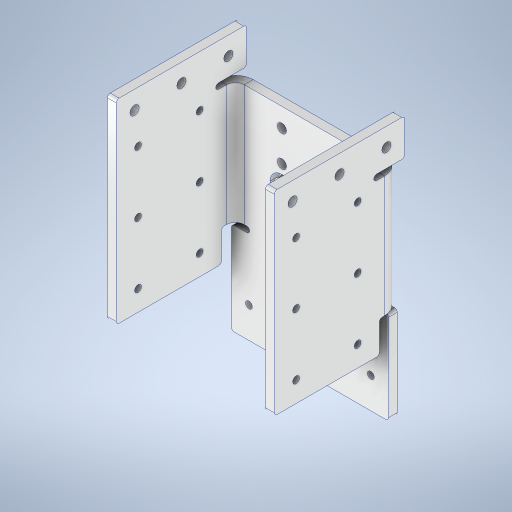
# Autodesk Inventor part: Printhead Baseplate
Saved by Autodesk Inventor 2024 (Build 280153000, 153)
## iProperties
Created: 2025-01-03
Part Number: Printhead Baseplate
Material: Aluminum 6061
Document SubType Name: Sheet Metal
Designer: Ishaan
Density: 2.7 g/cm^3
Sheet Metal Rule: SendCutSend_1-8_Alu
Appearance: Aluminum - Flat
Flat Pattern Width: 13.9913 cm
Flat Pattern Length: 9.325 cm
Flat Pattern Area: 130.469 cm^2
Sheet Metal Width: 139.913 mm
Sheet Metal Length: 93.250 mm
Sheet Metal Area: 13046.921 mm^2
Author: Ishaan
Autodesk Inventor part; units mm, degrees
ref_plane "YZ Plane" through (0, 0, 0) normal (1, 0, 0) x (0, 1, 0)
ref_plane "XZ Plane" through (0, 0, 0) normal (0, 1, 0) x (-1, 0, 0)
ref_plane "XY Plane" through (0, 0, 0) normal (0, 0, 1) x (1, 0, 0)
sketch "Sketch1" plane through (0, 0, 0) normal (0, 0, 1) x (1, 0, 0)
  line L0 (28, -13.5) -> (-28, -13.5)
  line L1 (-28, -13.5) -> (-28, 13.5)
  line L2 (-28, 13.5) -> (28, 13.5)
  line L3 (28, 13.5) -> (28, -13.5)
  line L4 (28, -13.5) -> (-28, 13.5) construction
  line L5 (-28, -13.5) -> (28, 13.5) construction
  line L6 (-28, -13.5) -> (28, -13.5)
  line L7 (28, -13.5) -> (28, -46.5)
  line L8 (28, -46.5) -> (-28, -46.5)
  line L9 (-28, -46.5) -> (-28, -13.5)
  line L10 (10, -10) -> (-10, -10) construction
  line L11 (-10, -10) -> (-10, 10) construction
  line L12 (-10, 10) -> (10, 10) construction
  line L13 (10, 10) -> (10, -10) construction
  line L14 (10, -10) -> (-10, 10) construction
  line L15 (-10, -10) -> (10, 10) construction
  line L16 (28, -47) -> (-28, -47) construction
  line L17 (-28, -47) -> (-28, -17) construction
  line L18 (-28, -17) -> (28, -17) construction
  line L19 (28, -17) -> (28, -47) construction
  line L20 (28, -47) -> (-28, -17) construction
  line L21 (-28, -47) -> (28, -17) construction
  circle A0 centre (0, -32) radius 11 construction
  circle A1 centre (0, -32) radius 8 construction
  line L22 (5.6569, -37.6569) -> (-5.6569, -37.6569) construction
  line L23 (-5.6569, -37.6569) -> (-5.6569, -26.3431) construction
  line L24 (-5.6569, -26.3431) -> (5.6569, -26.3431) construction
  line L25 (5.6569, -26.3431) -> (5.6569, -37.6569) construction
  line L26 (5.6569, -37.6569) -> (-5.6569, -26.3431) construction
  line L27 (-5.6569, -37.6569) -> (5.6569, -26.3431) construction
  line L28 (-21.75, -32) -> (21.75, -32) construction
  line L29 (16, -16) -> (-16, -16)
  line L30 (-16, -16) -> (-16, 16)
  line L31 (-16, 16) -> (16, 16)
  line L32 (16, 16) -> (16, -16)
  line L33 (16, -16) -> (-16, 16) construction
  line L34 (-16, -16) -> (16, 16) construction
  line L35 (16, -47) -> (-16, -47) construction
  line L36 (-16, -47) -> (-16, -17) construction
  line L37 (-16, -17) -> (16, -17) construction
  line L38 (16, -17) -> (16, -47) construction
  line L39 (16, -47) -> (-16, -17) construction
  line L40 (-16, -47) -> (16, -17) construction
  line L41 (13, -38.5) -> (-13, -38.5) construction
  line L42 (-13, -38.5) -> (-13, -25.5) construction
  line L43 (-13, -25.5) -> (13, -25.5) construction
  line L44 (13, -25.5) -> (13, -38.5) construction
  line L45 (13, -38.5) -> (-13, -25.5) construction
  line L46 (-13, -38.5) -> (13, -25.5) construction
  line L47 (28, -21) -> (-28, -21)
  line L48 (-28, -21) -> (-28, -43)
  line L49 (-28, -43) -> (28, -43)
  line L50 (28, -43) -> (28, -21)
  line L51 (28, -21) -> (-28, -43) construction
  line L52 (-28, -21) -> (28, -43) construction
  line L53 (-28, 13.5) -> (28, 13.5)
  line L54 (28, 13.5) -> (28, 35.25)
  line L55 (28, 35.25) -> (-28, 35.25)
  line L56 (-28, 35.25) -> (-28, 13.5)
  point P0 (0, 0)
  point P1 (-16, 13.5)
  point P2 (16, 13.5)
  point P3 (-28, -43)
  point P4 (28, -43)
  dimension "d8" = 16
  dimension "d0" = 56
  dimension "d1" = 27
  dimension "d2" = 60
  dimension "d3" = 20
  dimension "d4" = 20
  dimension "d5" = 30
  dimension "d6" = 32
  dimension "d7" = 22
  dimension "d9" = 43.5
  dimension "d32" = 32
  dimension "d33" = 32
  dimension "d41" = 32
  dimension "d42" = 26
  dimension "d43" = 13
  dimension "d61" = 22
  dimension "d73" = 35.25
  constraints: 114 end point, 20 parallel, 17 midpoint, 16 coincident, 11 horizontal, 11 perpendicular, 3 collinear, 2 point on line, 1 centre point, 1 vertical alignment, 3 other
  measures "d0" distance of L1.end L2.end
  measures "d1" distance of L0.end L1.end
  measures "d2" distance between parallel lines of L8 L2
  measures "d3" distance of L11.end L12.end
  measures "d4" distance of L10.end L11.end
  measures "d5" distance of L16.end L17.end
  measures "d6" distance of point (0, -32) point (0, 0)
  measures "d7" diameter of A0
  measures "d9" distance of L28.start L28.end
  measures "d32" distance of L30.end L31.end
  measures "d33" distance of L29.end L30.end
  measures "d41" distance of L36.end L37.end
  measures "d42" distance of L42.end L43.end
  measures "d43" distance of L41.end L42.end
  measures "d61" distance between parallel lines of L49 L47
  measures "d73" distance from line of L55 point (0, 0)
sketch "Sketch15" plane through (0, 0, 0) normal (0, 0, -1) x (-1, 0, 0)
  arc A0 (-13, -10) -> (-10, -13) centre (-10, -10) ccw projected
  line L0 (-10, -13) -> (10, -13) projected
  arc A1 (10, -13) -> (13, -10) centre (10, -10) ccw projected
  line L1 (13, -10) -> (13, 10) projected
  arc A2 (13, 10) -> (10, 13) centre (10, 10) ccw projected
  line L2 (10, 13) -> (8.25, 13) projected
  arc A3 (8.25, 14.5) -> (8.25, 13) centre (8.25, 13.75) ccw projected
  line L3 (8.25, 14.5) -> (10, 14.5) projected
  arc A4 (14.5, 10) -> (10, 14.5) centre (10, 10) ccw projected
  line L4 (14.5, 10) -> (14.5, -10) projected
  arc A5 (10, -14.5) -> (14.5, -10) centre (10, -10) ccw projected
  line L5 (10, -14.5) -> (-10, -14.5) projected
  arc A6 (-14.5, -10) -> (-10, -14.5) centre (-10, -10) ccw projected
  line L6 (-14.5, -10) -> (-14.5, 10) projected
  arc A7 (-10, 14.5) -> (-14.5, 10) centre (-10, 10) ccw projected
  line L7 (-10, 14.5) -> (-8.25, 14.5) projected
  arc A8 (-8.25, 13) -> (-8.25, 14.5) centre (-8.25, 13.75) ccw projected
  line L8 (-8.25, 13) -> (-10, 13) projected
  arc A9 (-10, 13) -> (-13, 10) centre (-10, 10) ccw projected
  line L9 (-13, 10) -> (-13, -10) projected
  arc A10 (9.25, 48.736) -> (7.25, 50.736) centre (7.25, 48.736) ccw projected
  line L10 (-7.25, 50.736) -> (7.25, 50.736) projected
  arc A11 (-7.25, 50.736) -> (-9.25, 48.736) centre (-7.25, 48.736) ccw projected
  line L11 (-9.25, 48.736) -> (-9.25, 39.736) projected
  arc A12 (-11.25, 37.736) -> (-9.25, 39.736) centre (-11.25, 39.736) ccw projected
  line L12 (-11.25, 37.736) -> (-23.45, 37.736) projected
  line L13 (-23.45, 37.736) -> (-23.45, -8) projected
  line L14 (-23.45, -8) -> (-22.5, -8) projected
  arc A13 (-22.5, -10) -> (-22.5, -8) centre (-22.5, -9) ccw projected
  line L15 (-22.5, -10) -> (-26, -10) projected
  arc A14 (-26, -10) -> (-28, -12) centre (-26, -12) ccw projected
  line L16 (-28, -41) -> (-28, -12) projected
  arc A15 (-28, -41) -> (-26, -43) centre (-26, -41) ccw projected
  line L17 (26, -43) -> (-26, -43) projected
  arc A16 (26, -43) -> (28, -41) centre (26, -41) ccw projected
  line L18 (28, -12) -> (28, -41) projected
  arc A17 (28, -12) -> (26, -10) centre (26, -12) ccw projected
  line L19 (26, -10) -> (22.5, -10) projected
  arc A18 (22.5, -8) -> (22.5, -10) centre (22.5, -9) ccw projected
  line L20 (22.5, -8) -> (23.45, -8) projected
  line L21 (23.45, -8) -> (23.45, 37.736) projected
  line L22 (23.45, 37.736) -> (11.25, 37.736) projected
  arc A19 (9.25, 39.736) -> (11.25, 37.736) centre (11.25, 39.736) ccw projected
  line L23 (9.25, 39.736) -> (9.25, 48.736) projected
  circle A20 centre (10, 10) radius 1.65 projected
  circle A21 centre (10, -10) radius 1.65 projected
  circle A22 centre (-10, 10) radius 1.65 projected
  circle A23 centre (-10, -10) radius 1.65 projected
  circle A24 centre (5.6569, -26.3431) radius 1.35 projected
  circle A25 centre (-5.6569, -26.3431) radius 1.35 projected
  circle A26 centre (-5.6569, -37.6569) radius 1.35 projected
  circle A27 centre (5.6569, -37.6569) radius 1.35 projected
  circle A28 centre (21.75, -32) radius 1.2295 projected
  circle A29 centre (-21.75, -32) radius 1.2295 projected
  circle A30 centre (0, -32) radius 2.15 projected
  circle A31 centre (10, 28.5) radius 1.65 projected
  circle A32 centre (-10, 28.5) radius 1.65 projected
  circle A33 centre (-10, 17.5) radius 1.65 projected
  circle A34 centre (10, 17.5) radius 1.65 projected
  circle A35 centre (-6, 39.736) radius 1.65 projected
  circle A36 centre (6, 39.736) radius 1.65 projected
  circle A37 centre (6, 47.736) radius 1.65 projected
  circle A38 centre (-6, 47.736) radius 1.65 projected
  circle A39 centre (0, -32) radius 11
  point P0 (0, 0)
  dimension "d145" = 22
  constraints: 1 centre point, 1 coincident
  measures "d145" diameter of A39
extrude "Plate1" add sketch "Sketch1" along normal blind 3.175 contours L7 L47 L9 L0 L30 L29 L32 | L0 L32 L2 L3 | L32 L29 L30 L0 | L0 L30 L2 L32 | L2 L32 L31 L30 L56 L55 L54 | L7 L49 L9 L47 | L0 L1 L2 L30 | L2 L30 L31 L32
hole "Hole1" at (-10, 10, 0) at (-10, -10, 0) at (10, 10, 0) at (10, -10, 0) direction (0, 0, 1) diameter 3.3 end through all
hole "Hole2" at (-5.6569, -26.3431, 0) at (5.6569, -26.3431, 0) at (5.6569, -37.6569, 0) at (-5.6569, -37.6569, 0) direction (0, 0, 1) diameter 2.7 end through all
hole "Hole3" at (-21.75, -32, 0) at (21.75, -32, 0) direction (0, 0, 1) diameter 2.459 end through all thread size "M3x0.5" class "6H" standard "ANSI Metric M Profile"
hole "Hole4" at (0, -32, 0) direction (0, 0, 1) diameter 4.3 end through all
sketch "Sketch2" plane through (0, 0, 3.175) normal (0, 0, 1) x (1, 0, 0)
  line L0 (10, 17.5) -> (-10, 17.5) construction
  line L1 (-10, 17.5) -> (-10, 28.5) construction
  line L2 (-10, 28.5) -> (10, 28.5) construction
  line L3 (10, 28.5) -> (10, 17.5) construction
  line L4 (10, 17.5) -> (-10, 28.5) construction
  line L5 (-10, 17.5) -> (10, 28.5) construction
  point P0 (0, 0)
  point P1 (0, 23)
  dimension "d51" = 20
  dimension "d52" = 11
  dimension "d137" = 23
  constraints: 12 end point, 4 coincident, 2 midpoint, 2 parallel, 1 horizontal, 1 perpendicular, 1 vertical alignment
  measures "d51" distance of L1.end L2.end
  measures "d52" distance of L0.end L1.end
  measures "d137" distance of point (0, 0) point (0, 23)
hole "Hole6" at (-10, 28.5, 3.175) at (10, 28.5, 3.175) at (10, 17.5, 3.175) at (-10, 17.5, 3.175) direction (0, 0, -1) diameter 3.3 end through all
sketch "Sketch8" plane through (0, 0, 3.175) normal (0, 0, 1) x (1, 0, 0)
  circle A0 centre (-10, 17.5) radius 1.65 construction
  circle A1 centre (10, 17.5) radius 1.65 construction
  circle A2 centre (10, 28.5) radius 1.65 construction
  circle A3 centre (-10, 28.5) radius 1.65 construction
  circle A4 centre (0, -32) radius 2.15 construction
  circle A5 centre (21.75, -32) radius 1.2295 construction
  circle A6 centre (-21.75, -32) radius 1.2295 construction
  circle A7 centre (-5.6569, -37.6569) radius 1.35 construction
  circle A8 centre (5.6569, -37.6569) radius 1.35 construction
  circle A9 centre (5.6569, -26.3431) radius 1.35 construction
  circle A10 centre (-5.6569, -26.3431) radius 1.35 construction
  circle A11 centre (10, -10) radius 1.65 construction
  circle A12 centre (10, 10) radius 1.65 construction
  circle A13 centre (-10, -10) radius 1.65 construction
  circle A14 centre (-10, 10) radius 1.65 construction
  line L0 (-28, -43) -> (-28, 35.25) projected
  line L1 (28, -43) -> (-28, -43) projected
  line L2 (28, 35.25) -> (28, -43) projected
  line L3 (-28, 35.25) -> (28, 35.25) projected
  line L4 (-28, -9) -> (-22.5, -9) construction
  line L5 (-28, -10) -> (-22.5, -10)
  line L6 (-22.5, -8) -> (-28, -8)
  arc A15 (-28, -8) -> (-28, -10) centre (-28, -9) ccw
  arc A16 (-22.5, -10) -> (-22.5, -8) centre (-22.5, -9) ccw
  line L7 (28, -9) -> (22.5, -9) construction
  line L8 (28, -8) -> (22.5, -8)
  line L9 (22.5, -10) -> (28, -10)
  arc A17 (28, -10) -> (28, -8) centre (28, -9) ccw
  arc A18 (22.5, -8) -> (22.5, -10) centre (22.5, -9) ccw
  line L10 (-22.5, -9) -> (22.5, -9) construction
  line L11 (-26.625, -8) -> (26.625, -8)
  line L12 (26.625, -8) -> (26.625, 35.25)
  line L13 (26.625, 35.25) -> (-26.625, 35.25)
  line L14 (-26.625, 35.25) -> (-26.625, -8)
  line L15 (-26.625, -8) -> (-29.8, -8) construction
  line L16 (-29.8, -8) -> (-29.8, 35.25) construction
  line L17 (-29.8, 35.25) -> (-26.625, 35.25) construction
  line L18 (-26.625, 35.25) -> (-26.625, -8) construction
  line L19 (26.625, -8) -> (29.8, -8) construction
  line L20 (29.8, -8) -> (29.8, 35.25) construction
  line L21 (29.8, 35.25) -> (26.625, 35.25) construction
  line L22 (26.625, 35.25) -> (26.625, -8) construction
  point P0 (0, 0)
  point P1 (-25.25, -9)
  point P2 (25.25, -9)
  point P3 (0, 35.25)
  point P4 (28, -10)
  point P5 (28, -10)
  point P6 (28, -8)
  point P7 (-28, -8)
  point P8 (-28, -10)
  dimension "d104" = 2
  dimension "d105" = 23
  dimension "d106" = 45
  dimension "d107" = 53.25
  dimension "d108" = 3.175
  constraints: 42 end point, 8 parallel, 8 point on circle, 8 tangent, 6 point on line, 5 perpendicular, 4 centre point, 3 collinear, 3 horizontal, 3 midpoint, 1 equal radius, 1 vertical alignment
  measures "d104" diameter of A16
  measures "d105" distance from line of L4 A4.centre
  measures "d106" distance of L4.end L7.end
  measures "d107" distance between parallel lines of L12 L14
  measures "d108" distance of L16.end L17.end
extrude "Extrusion2" cut sketch "Sketch8" against normal up to surface (3.175 mm away) contours L0 L6 A16 L5 | L0 L3 L14 L6 | L9 A18 L8 L2 | L8 L12 L3 L2
sketch "Sketch9" plane through (-26.625, -8, 3.175) normal (-1, 0, 0) x (0, -1, 0)
  line L0 (-43.25, 0) -> (0, 0)
  line L1 (0, 0) -> (0, 5)
  line L2 (0, 5) -> (-43.25, 5)
  line L3 (-43.25, 5) -> (-43.25, 0)
  constraints: 6 end point, 1 horizontal, 1 perpendicular, 1 vertical
edge flange "Flange3" height 5 angle 90 thickness 3.175 bend radius 3.175 thickness toward (-1, 0, 0) relief straight relief width 2 relief depth 1.5875 corner gap 3.175 corner form 0 edges at (-26.625, 13.625, 3.175) (26.625, 13.625, 3.175) wall of the first edge with corners at (-26.625, 35.25, 3.175) (-26.625, -8, 3.175) (-26.625, -8, 8.175) (-26.625, 35.25, 8.175)
bend "Bend3"
corner "Corner3"
fillet "Fillet2" radius 1 4 edges at (28, -10, 1.5875) (28, -43, 1.5875) (-28, -10, 1.5875) (-28, -43, 1.5875)
sketch "Sketch13" plane through (0, 0, 3.175) normal (0, 0, 1) x (1, 0, 0)
  circle A0 centre (-10, 10) radius 1.65 projected
  circle A1 centre (10, 10) radius 1.65 projected
  circle A2 centre (10, -10) radius 1.65 projected
  circle A3 centre (-10, -10) radius 1.65 projected
  circle A4 centre (-10, 10) radius 3 construction
  circle A5 centre (-10, -10) radius 3 construction
  circle A6 centre (10, -10) radius 3 construction
  circle A7 centre (10, 10) radius 3 construction
  line L0 (10, -13) -> (-10, -13)
  line L1 (-13, -10) -> (-13, 10)
  line L2 (-10, 13) -> (10, 13)
  line L3 (13, 10) -> (13, -10)
  line L4 (13, -13) -> (-13, 13) construction
  line L5 (-13, -13) -> (13, 13) construction
  arc A8 (-10, 13) -> (-13, 10) centre (-10, 10) ccw
  arc A9 (13, 10) -> (10, 13) centre (10, 10) ccw
  arc A10 (10, -13) -> (13, -10) centre (10, -10) ccw
  arc A11 (-13, -10) -> (-10, -13) centre (-10, -10) ccw
  line L6 (10, 14.25) -> (-10, 14.25)
  arc A12 (-10, 14.25) -> (-14.25, 10) centre (-10, 10) ccw
  line L7 (-14.25, 10) -> (-14.25, -10)
  arc A13 (-14.25, -10) -> (-10, -14.25) centre (-10, -10) ccw
  line L8 (-10, -14.25) -> (10, -14.25)
  arc A14 (10, -14.25) -> (14.25, -10) centre (10, -10) ccw
  line L9 (14.25, -10) -> (14.25, 10)
  arc A15 (14.25, 10) -> (10, 14.25) centre (10, 10) ccw
  line L10 (7.5, -14.25) -> (-7.5, -14.25)
  line L11 (-7.5, -14.25) -> (-7.5, 14.25)
  line L12 (-7.5, 14.25) -> (7.5, 14.25)
  line L13 (7.5, 14.25) -> (7.5, -14.25)
  line L14 (7.5, -14.25) -> (-7.5, 14.25) construction
  line L15 (-7.5, -14.25) -> (7.5, 14.25) construction
  circle A16 centre (-8.125, 13.625) radius 0.625
  circle A17 centre (8.125, 13.625) radius 0.625
  point P0 (0, 0)
  point P1 (0, 0)
  point P2 (-7.5, 13)
  point P3 (7.5, 14.25)
  point P4 (7.5, 13)
  point P5 (-8.125, 13)
  point P6 (-8.125, 14.25)
  point P7 (8.125, 14.25)
  point P8 (8.125, 13)
  dimension "d138" = 6
  dimension "d140" = 1.25
  dimension "d141" = 15
  constraints: 32 end point, 16 point on circle, 15 tangent, 14 centre point, 9 point on line, 6 coincident, 6 equal radius, 6 parallel, 4 midpoint, 3 perpendicular, 2 horizontal, 7 other
  measures "d138" diameter of A4
  measures "d140" distance between parallel lines of L2 L6
  measures "d141" distance of L11.end L12.end
extrude "Extrusion6" cut sketch "Sketch13" against normal through all contours A10 L3 A9 L2 A17 L6 A15 L9 A14 L8 L13 L0 | L13 L8 L11 L0 | L11 L8 A13 L7 A12 L6 A16 L2 A8 L1 A11 L0 | A17 | A16
sketch "Sketch17" plane through (26.625, -8, 8.175) normal (-1, 0, 0) x (0, 0, 1)
  line L0 (37.5, 58.25) -> (-9, 58.25)
  line L1 (-9, 58.25) -> (-9, 45.25)
  line L2 (-9, 45.25) -> (37.5, 45.25)
  line L3 (37.5, 45.25) -> (37.5, 58.25)
  line L4 (0, 0) -> (0, 43.25) projected
  line L5 (0, 43.25) -> (2, 43.25)
  line L6 (2, 43.25) -> (2, 45.25)
  line L7 (2, 45.25) -> (0, 45.25)
  line L8 (0, 45.25) -> (0, 43.25)
  circle A0 centre (1, 44.25) radius 1
  circle A1 centre (33.8129, -20.85) radius 1.5 construction
  line L9 (-1.825, 43.25) -> (-1.825, 0) projected
  line L10 (-1.825, 43.25) -> (0, 43.25) projected
  line L11 (-1.825, 0) -> (0, 0) projected
  line L12 (37.5, 45.25) -> (0, 45.25)
  line L13 (0, 45.25) -> (0, -11.35)
  line L14 (0, -11.35) -> (37.5, -11.35)
  line L15 (37.5, -11.35) -> (37.5, 45.25)
  circle A2 centre (33.8129, -20.85) radius 9.5
  line L16 (-10, -2) -> (-10, 58) construction
  line L17 (45.709, 60) -> (-8, 60) construction
  point P0 (-8.175, 8)
  point P1 (1, 45.25)
  point P2 (1, 43.25)
  point P3 (0, 43.25)
  point P4 (2, 44.25)
  point P5 (0, 45.25)
  dimension "d154" = 0
  dimension "d153" = 46.5
  dimension "d155" = 2
  dimension "d156" = 2
  dimension "d168" = 19
  dimension "d169" = 1.75
  dimension "d170" = 1
  constraints: 28 end point, 6 horizontal, 6 parallel, 5 point on line, 4 tangent, 3 centre point, 3 perpendicular, 3 vertical, 1 coincident, 1 collinear, 13 other
  measures "d153" distance of point (37.5, 58.25) point (-9, 58.25)
  measures "d155" distance of L4.end L5.end
  measures "d156" distance between parallel lines of L2 L5
  measures "d168" diameter of A2
  measures "d169" distance between parallel lines of L0 L17
  measures "d170" distance between parallel lines of L1 L16
extrude "Extrusion9" add sketch "Sketch17" against normal up to surface (3.175 mm away) contours L3 L2 L1 L0 | L15 L14 L13 L4 L5 L6 L2 | L6 A0 L2 | L6 L5 A0
mirror "Mirror4" about plane through (0, 0, 0) normal (1, 0, 0) of "Extrusion9"
sketch "Sketch19" plane through (-29.8, -8, 6.35) normal (-1, 0, 0) x (0, 0, 1)
  line L0 (0, 43.25) -> (0, 0) projected
  line L1 (1.825, 0) -> (0, 0) projected
  line L2 (1.825, -11.35) -> (1.825, 0) projected
  line L3 (39.325, -11.35) -> (1.825, -11.35) projected
  line L4 (39.325, 58.25) -> (39.325, -11.35) projected
  line L5 (-7.175, 58.25) -> (39.325, 58.25) projected
  line L6 (-7.175, 45.25) -> (-7.175, 58.25) projected
  line L7 (2.825, 45.25) -> (-7.175, 45.25) projected
  arc A0 (2.825, 43.25) -> (2.825, 45.25) centre (2.825, 44.25) ccw projected
  line L8 (0, 43.25) -> (2.825, 43.25) projected
  line L9 (39.325, 45.25) -> (-7.175, 45.25) construction
  line L10 (-7.175, 45.25) -> (-7.175, 58.25) construction
  line L11 (-7.175, 58.25) -> (39.325, 58.25) construction
  line L12 (39.325, 58.25) -> (39.325, 45.25) construction
  line L13 (39.325, 45.25) -> (-7.175, 58.25) construction
  line L14 (-7.175, 45.25) -> (39.325, 58.25) construction
  line L15 (32.825, 51.75) -> (-0.675, 51.75) construction
  line L16 (-3.175, -34) -> (-3.175, -3) projected
  point P0 (-6.35, 8)
  point P1 (16.075, 51.75)
  point P2 (16.075, 51.75)
  point P3 (-6.35, -24)
  dimension "d172" = 6.5
  dimension "d173" = 6.5
  dimension "d193" = 75.75
  dimension "d194" = 19.25
  dimension "d195" = 33.5
  constraints: 14 end point, 3 coincident, 3 midpoint, 2 horizontal, 2 parallel, 1 perpendicular
  measures "d172" distance between parallel lines of L11 L15
  measures "d173" distance from line of L4 L15.start
  measures "d193" vertical distance of point (16.075, 51.75) point (-6.35, -24)
  measures "d194" distance from line of point (16.075, 51.75) L16
  measures "d195" distance of L15.start L15.end
hole "Hole8" at (-29.8, 43.75, 39.175) at (-29.8, 43.75, 22.425) at (-29.8, 43.75, 5.675) direction (1, 0, 0) diameter 3.3 end through all
sketch "Sketch21" plane through (-29.8, -8, 6.35) normal (-1, 0, 0) x (0, 0, 1)
  circle A0 centre (-0.675, 51.75) radius 1.65 projected
  circle A1 centre (16.075, 51.75) radius 1.65 projected
  circle A2 centre (32.825, 51.75) radius 1.65 projected
  line L0 (0, 43.25) -> (0, 0) projected
  line L1 (1.825, 0) -> (0, 0) projected
  line L2 (1.825, -11.35) -> (1.825, 0) projected
  line L3 (39.325, -11.35) -> (1.825, -11.35) projected
  line L4 (39.325, 58.25) -> (39.325, -11.35) projected
  line L5 (-7.175, 58.25) -> (39.325, 58.25) projected
  line L6 (-7.175, 45.25) -> (-7.175, 58.25) projected
  line L7 (2.825, 45.25) -> (-7.175, 45.25) projected
  arc A3 (2.825, 43.25) -> (2.825, 45.25) centre (2.825, 44.25) ccw projected
  line L8 (0, 43.25) -> (2.825, 43.25) projected
  line L9 (9.575, -4) -> (31.575, -4)
  line L10 (31.575, -4) -> (31.575, 40)
  line L11 (31.575, 40) -> (9.575, 40)
  line L12 (9.575, 40) -> (9.575, -4)
  line L13 (9.575, -4) -> (31.575, 40) construction
  line L14 (31.575, -4) -> (9.575, 40) construction
  line L15 (-3.175, -34) -> (-3.175, -3) projected
  point P0 (-6.35, 8)
  point P1 (20.575, 18)
  point P2 (9.575, 18)
  point P3 (31.575, 18)
  point P4 (20.575, -11.35)
  point P5 (-6.35, -24)
  dimension "d181" = 22
  dimension "d182" = 44
  dimension "d183" = 10
  dimension "d191" = 42
  dimension "d192" = 23.75
  constraints: 12 end point, 5 midpoint, 4 coincident, 2 parallel, 1 horizontal, 1 perpendicular, 1 vertical alignment
  measures "d181" distance of L11.end L10.end
  measures "d182" distance of L10.end L9.end
  measures "d183" vertical distance of point (9.575, 18) point (-6.35, 8)
  measures "d191" vertical distance of point (20.575, 18) point (-6.35, -24)
  measures "d192" distance from line of point (20.575, 18) L15
hole "Hole9" at (-29.8, 32, 37.925) at (-29.8, 32, 15.925) at (-29.8, 10, 15.925) at (-29.8, 10, 37.925) at (-29.8, -12, 37.925) at (-29.8, -12, 15.925) direction (1, 0, 0) diameter 2.459 depth 3.175 tip angle 118 thread size "M3x0.5" class "6H" standard "ANSI Metric M Profile"
mirror "Mirror5" about plane through (0, 0, 0) normal (1, 0, 0) of "Hole9"
fillet "Fillet6" radius 1 12 edges at (-28.2125, -19.35, 8.175) (-28.2125, -19.35, 45.675) (28.2125, -19.35, 8.175) (-28.2125, 37.25, -0.825) (28.2125, 37.25, -0.825) (28.2125, -19.35, 45.675) (28.2125, 50.25, 45.675) (-28.2125, 50.25, 45.675) (-28.2125, 50.25, -0.825) (28.2125, 50.25, -0.825) (28.2125, -8, 8.175) (-28.2125, -8, 8.175)
equation "\"d16\" = Thickness"
equation "\"d59\" = Thickness"
equation "\"d10\" = Thickness"
equation "\"d111\" = BendReliefWidth"
equation "\"d112\" = BendReliefDepth"
equation "\"d113\" = MinimumRemnant"
equation "\"d114\" = TransitionRadius"
equation "\"d117\" = BendRadius"
equation "\"d118\" = CornerReliefSize"
equation "\"d119\" = GapSize"
equation "\"d120\" = JacobiRadiusSize"
equation "\"BendReliefDepth\" = 0.5 * Thickness"
equation "\"CornerReliefSize\" = 4 * Thickness"
equation "\"MinimumRemnant\" = 2 * Thickness"
equation "\"TransitionRadius\" = BendRadius"
equation "\"JacobiRadiusSize\" = BendRadius"
equation "\"Thickness\" = 3.175"
equation "\"BendReliefWidth\" = 2"
equation "\"BendRadius\" = 3.175"
equation "\"GapSize\" = 2"
body "Solid1"
